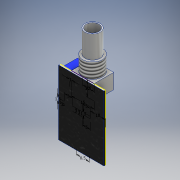
# Autodesk Inventor part: Ph Reader
Saved by Autodesk Inventor 2016 (Build 200138000, 138)
## iProperties
Created: 2016-05-08
Part Number: Ph Reader
Material: Generic
Document SubType Name: Modeling
Designer: Kenneth Daniel
Density: 1 g/cm^3
Appearance: Default
Author: Kenneth Daniel
Autodesk Inventor part; units mm, degrees
ref_plane "YZ Plane" through (0, 0, 0) normal (1, 0, 0) x (0, 1, 0)
ref_plane "XZ Plane" through (0, 0, 0) normal (0, 1, 0) x (-1, 0, 0)
ref_plane "XY Plane" through (0, 0, 0) normal (0, 0, 1) x (1, 0, 0)
sketch "Sketch1" plane through (0, 0, 0) normal (0, 1, 0) x (-1, 0, 0)
  line L0 (-15, 21.5) -> (-15, -21.5)
  line L1 (-15, -21.5) -> (15, -21.5)
  line L2 (15, -21.5) -> (15, 21.5)
  line L3 (15, 21.5) -> (-15, 21.5)
  line L4 (-15, 21.5) -> (15, -21.5) construction
  line L5 (-15, -21.5) -> (15, 21.5) construction
  point P0 (0, 0)
  dimension "d0" = 43
  dimension "d1" = 30
  constraints: 12 end point, 2 midpoint, 2 parallel, 1 perpendicular, 1 vertical
  measures "d0" distance of L0.start L0.end
  measures "d1" distance of L1.end L0.end
extrude "Extrusion1" add sketch "Sketch1" along normal blind 1
sketch "Sketch2" plane through (0, 1, 0) normal (0, 1, 0) x (1, 0, 0)
  line L0 (4.25, 16.6043) -> (4.25, 21.5)
  line L1 (4.25, 21.5) -> (-4.25, 21.5)
  line L2 (-4.25, 21.5) -> (-4.25, 16.6043)
  line L3 (-4.25, 16.6043) -> (4.25, 16.6043)
  line L4 (4.25, 16.6043) -> (-4.25, 21.5) construction
  line L5 (4.25, 21.5) -> (-4.25, 16.6043) construction
  line L6 (-15, 21.5) -> (-15, -21.5) construction
  line L7 (-15, 0) -> (-12, 0) construction
  line L8 (-12, 0) -> (-12, -1.5) construction
  line L9 (-12, -1.5) -> (-7, -1.5) construction
  line L10 (-7, -1.5) -> (-7, 1.5) construction
  line L11 (-12, -1.5) -> (-7, -1.5)
  line L12 (-7, -1.5) -> (-7, 1.5)
  line L13 (-7, 1.5) -> (-12, 1.5)
  line L14 (-12, 1.5) -> (-12, -1.5)
  line L15 (15, -21.5) -> (15, 21.5) projected
  line L16 (15, 0) -> (5, 0) construction
  line L17 (5, 0) -> (5, -1.5)
  line L18 (5, -1.5) -> (0, -1.5)
  line L19 (0, -1.5) -> (0, 1.5)
  line L20 (0, 1.5) -> (5, 1.5)
  line L21 (5, 1.5) -> (5, 0)
  line L22 (0, -21.5) -> (7.5, -21.5)
  line L23 (-15, -21.5) -> (15, -21.5) projected
  line L24 (7.5, -21.5) -> (7.5, -11.5)
  line L25 (7.5, -11.5) -> (-7.5, -11.5)
  line L26 (-7.5, -11.5) -> (-7.5, -21.5)
  line L27 (-7.5, -21.5) -> (7.5, -21.5)
  line L28 (-7.5, -11.5) -> (-8.5, -11.5) construction
  line L29 (-8.5, -11.5) -> (-13.5, -11.5)
  line L30 (-13.5, -11.5) -> (-13.5, -20.6777)
  line L31 (-13.5, -20.6777) -> (-8.5, -20.6777)
  line L32 (-8.5, -20.6777) -> (-8.5, -11.5)
  point P0 (0, 0)
  point P1 (0, 19.0521)
  dimension "d4" = 8.5
  dimension "d5" = 3
  dimension "d6" = 1.5
  dimension "d7" = 5
  dimension "d8" = 3
  dimension "d9" = 10
  dimension "d10" = 1.5
  dimension "d11" = 5
  dimension "d12" = 3
  dimension "d13" = 5
  dimension "d14" = 7.5
  dimension "d15" = 10
  dimension "d16" = 15
  dimension "d17" = 1
  constraints: 60 end point, 9 perpendicular, 6 parallel, 5 point on line, 4 horizontal, 4 midpoint, 3 vertical, 1 collinear
  measures "d4" distance of L1.end L0.end
  measures "d5" distance of L7.start L7.end
  measures "d6" distance of L7.end L8.end
  measures "d7" distance of L8.end L9.end
  measures "d8" distance of L9.end L10.end
  measures "d9" distance of L16.start L16.end
  measures "d10" distance of L16.end L17.end
  measures "d11" distance of L17.end L18.end
  measures "d12" distance of L18.end L19.end
  measures "d13" distance of L19.end L20.end
  measures "d14" distance of L22.start L22.end
  measures "d15" distance of L22.end L24.end
  measures "d16" distance of L24.end L25.end
  measures "d17" distance of L25.end L28.end
extrude "Extrusion2" add sketch "Sketch2" along normal blind 1 contours L14 L13 L12 L11 | L17 L18 L19 L20 L21
extrude "Extrusion3" add sketch "Sketch2" along normal blind 3 contours L3 L2 L1 L0
extrude "Extrusion4" add sketch "Sketch2" along normal blind 13 contours L23 L26 L25 L24 L22
extrude "Extrusion5" add sketch "Sketch2" along normal blind 10 contours L32 L31 L30 L29
sketch "Sketch3" plane through (0, 11, 0) normal (0, 1, 0) x (1, 0, 0)
  circle A0 centre (-12.491, -19.5006) radius 1.111
  point P0 (0, 0)
  constraints: 1 centre point
extrude "Extrusion6" add sketch "Sketch3" along normal blind 0.5
sketch "Sketch4" plane through (0, 14, 0) normal (0, 1, 0) x (1, 0, 0)
  line L0 (7.5, -11.5) -> (7.5, -21.5) construction
  line L1 (7.5, -11.5) -> (-7.5, -11.5) construction
  line L2 (7.5, -21.5) -> (-7.5, -11.5) construction
  line L3 (-7.5, -11.5) -> (-7.5, -21.5) construction
  line L4 (-15, -21.5) -> (15, -21.5) construction
  line L5 (-7.5, -21.5) -> (7.5, -11.5) construction
  line L6 (5.8773, -20.4182) -> (-5.8773, -20.4182) construction
  line L7 (-5.8773, -20.4182) -> (-5.8773, -14.4182) construction
  line L8 (-5.8773, -14.4182) -> (5.8773, -14.4182) construction
  line L9 (5.8773, -14.4182) -> (5.8773, -20.4182) construction
  line L10 (5.8773, -20.4182) -> (-5.8773, -20.4182)
  line L11 (-5.8773, -20.4182) -> (-5.8773, -14.4182)
  line L12 (-5.8773, -14.4182) -> (5.8773, -14.4182)
  line L13 (5.8773, -14.4182) -> (5.8773, -20.4182)
  point P0 (0, 0)
  dimension "d28" = 6
  constraints: 22 end point, 4 perpendicular, 3 parallel, 3 point on line, 1 horizontal, 1 vertical
  measures "d28" distance of L6.end L7.end
extrude "Extrusion7" cut sketch "Sketch4" against normal blind 2
sketch "Sketch5" plane through (15, 0, -21.5) normal (0, 0, -1) x (-1, 0, 0)
  line L0 (10.75, 1) -> (10.75, 4) projected
  line L1 (19.25, 1) -> (19.25, 4) projected
  line L2 (10.75, 1) -> (19.25, 1)
  line L3 (10.75, 1) -> (19.25, 4) construction
  line L4 (19.25, 1) -> (10.75, 4) construction
  line L5 (12.5, 1.6176) -> (12.5, 3.3824)
  line L6 (12.5, 1.6176) -> (17.5, 1.6176)
  line L7 (17.5, 1.6176) -> (17.5, 3.3824)
  line L8 (17.5, 3.3824) -> (12.5, 3.3824)
  point P0 (15, 0)
  constraints: 14 end point, 3 perpendicular, 3 point on line, 1 horizontal, 1 vertical
extrude "Extrusion8" cut sketch "Sketch5" against normal blind 2
sketch "Sketch6" plane through (-15, 0, 21.5) normal (0, 0, 1) x (1, 0, 0)
  line L0 (0, 0) -> (30, 0) projected
  line L1 (30, 0) -> (30, 1) projected
  line L2 (22.5, 1) -> (30, 1) projected
  line L3 (22.5, 1) -> (22.5, 14) projected
  line L4 (7.5, 14) -> (22.5, 14) projected
  line L5 (7.5, 1) -> (7.5, 14) projected
  line L6 (0, 1) -> (7.5, 1) projected
  line L7 (0, 0) -> (0, 1) projected
  circle A0 centre (15, 7.5) radius 6.5
  point P0 (15, 0)
  constraints: 1 centre point
extrude "Extrusion9" add sketch "Sketch6" along normal blind 10 contours A0
sketch "Sketch7" plane through (0, 7.5, 31.5) normal (0, 0, 1) x (1, 0, 0)
  circle A0 centre (0, 0) radius 5
  point P0 (0, -7.5)
  dimension "d35" = 10
  constraints: 1 centre point
  measures "d35" diameter of A0
extrude "Extrusion10" add sketch "Sketch7" along normal blind 15
thread "Thread1" size "M14x2" class "6g" standard "ANSI Metric M Profile" full length
sketch "Sketch8" plane through (0, 7.5, 46.5) normal (0, 0, 1) x (1, 0, 0)
  circle A0 centre (0, 0) radius 5 projected
  circle A1 centre (0, 0) radius 4.25
  point P0 (0, -7.5)
  dimension "d40" = 0.75
  constraints: 1 centre point
  measures "d40" radial gap between concentric circles of A0 A1
extrude "Extrusion11" cut sketch "Sketch8" against normal blind 15 contours A1
body "Solid1"
